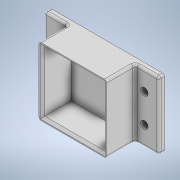
# Autodesk Inventor part: trypsinHolder
Saved by Autodesk Inventor 2020 (Build 240168000, 168)
## iProperties
Created: 2023-03-07
Part Number: trypsinHolder
Material: Generic
Document SubType Name: Modeling
Designer: DSOB
Density: 1 g/cm^3
Appearance: Default
Author: DSOB
Autodesk Inventor part; units mm, degrees
ref_plane "YZ Plane" through (0, 0, 0) normal (1, 0, 0) x (0, 1, 0)
ref_plane "XZ Plane" through (0, 0, 0) normal (0, 1, 0) x (-1, 0, 0)
ref_plane "XY Plane" through (0, 0, 0) normal (0, 0, 1) x (1, 0, 0)
sketch "Sketch1" plane through (0, 0, 0) normal (0, 0, 1) x (1, 0, 0)
  line L0 (0, 0) -> (100, 0)
  line L1 (100, 0) -> (100, 59)
  line L2 (100, 59) -> (0, 59)
  line L3 (0, 59) -> (0, 0)
  dimension "d0" = 100
  dimension "d1" = 59
  constraints: 8 end point, 2 parallel, 1 horizontal, 1 perpendicular
  measures "d0" distance of L1.end L2.end
  measures "d1" distance of L0.end L1.end
extrude "Extrusion1" add sketch "Sketch1" along normal blind 5
sketch "Sketch2" plane through (0, 0, 5) normal (0, 0, 1) x (1, 0, 0)
  line L0 (0, 0) -> (100, 0) projected
  line L1 (100, 59) -> (0, 59) projected
  line L2 (79.5, 0) -> (20.5, 0)
  line L3 (20.5, 0) -> (20.5, 59)
  line L4 (20.5, 59) -> (79.5, 59)
  line L5 (79.5, 59) -> (79.5, 0)
  line L6 (76.5, 3) -> (23.5, 3)
  line L7 (23.5, 3) -> (23.5, 56)
  line L8 (23.5, 56) -> (76.5, 56)
  line L9 (76.5, 56) -> (76.5, 3)
  line L10 (100, 0) -> (100, 59) projected
  point P0 (79.5, 59)
  point P1 (20.5, 0)
  dimension "d4" = 59
  dimension "d5" = 53
  dimension "d6" = 3
  dimension "d7" = 3
  dimension "d8" = 3
  dimension "d9" = 20.5
  constraints: 16 end point, 4 parallel, 2 horizontal, 2 perpendicular, 2 point on line
  measures "d4" distance between parallel lines of L3 L5
  measures "d5" distance of L6.start L6.end
  measures "d6" distance between parallel lines of L3 L7
  measures "d7" distance between parallel lines of L0 L6
  measures "d8" distance between parallel lines of L1 L8
  measures "d9" distance between parallel lines of L5 L10
extrude "Extrusion2" add sketch "Sketch2" along normal blind 25 contours L3 L1 L5 L0
chamfer "Chamfer1" distance 2 angle 45 1 edges at (50, 3, 30)
chamfer "Chamfer2" distance 2 angle 45 1 edges at (76.5, 29.5, 30)
chamfer "Chamfer3" distance 2 angle 45 2 edges at (50, 56, 30) (23.5, 29.5, 30)
sketch "Sketch3" plane through (0, 0, 5) normal (0, 0, 1) x (1, 0, 0)
  circle A0 centre (87.5, 17) radius 3.25
  circle A1 centre (87.5, 42) radius 3.25
  line L0 (100, 0) -> (100, 59) projected
  line L1 (0, 0) -> (100, 0) projected
  line L2 (50, -16.6248) -> (50, 70.7208)
  line L3 (0, 59) -> (0, 0) projected
  circle A2 centre (12.5, 17) radius 3.25
  circle A3 centre (12.5, 42) radius 3.25
  point P0 (79.5, 0)
  dimension "d21" = 6.5
  dimension "d22" = 6.5
  dimension "d23" = 12.5
  dimension "d24" = 12.5
  dimension "d25" = 25
  dimension "d26" = 17
  dimension "d27" = 50
  constraints: 4 centre point, 2 end point, 2 symmetric about line, 1 vertical, 2 other
  measures "d21" diameter of A0
  measures "d22" diameter of A1
  measures "d23" distance from line of L0 A0.centre
  measures "d24" distance from line of L0 A1.centre
  measures "d25" distance of A0.centre A1.centre
  measures "d26" distance from line of L1 A0.centre
  measures "d27" distance between parallel lines of L3 L2
extrude "Extrusion3" cut sketch "Sketch3" against normal blind 60
fillet "Fillet1" radius 2 2 edges at (20.5, 29.5, 5) (79.5, 29.5, 5)
fillet "Fillet2" radius 2 2 edges at (0, 29.5, 5) (100, 29.5, 5)
fillet "Fillet3" radius 2 20 edges at (20.5, 0, 18.5) (19.9142, 0, 5.5858) (10.25, 0, 5) (0.5858, 0, 4.4142) (0, 0, 1.5) (79.5, 0, 18.5) (80.0858, 0, 5.5858) (89.75, 0, 5) (99.4142, 0, 4.4142) (100, 0, 1.5) (79.5, 59, 18.5) (80.0858, 59, 5.5858) (89.75, 59, 5) (99.4142, 59, 4.4142) (100, 59, 1.5) (20.5, 59, 18.5) (19.9142, 59, 5.5858) (10.25, 59, 5) (0.5858, 59, 4.4142) (0, 59, 1.5)
body "Solid1"
